Autodesk Fusion 360 part; units mm, degrees
(part 3 of 8)
  line L1878 (6.35, -70.8501) -> (9.35, -70.8501)
  line L1879 (9.35, -70.8501) -> (9.35, -67.8501)
  line L1880 (9.35, -67.8501) -> (6.35, -67.8501)
  line L1881 (6.35, -67.8501) -> (6.35, -64.8501)
  line L1882 (6.35, -64.8501) -> (9.35, -64.8501)
  line L1883 (9.35, -64.8501) -> (9.35, -61.8501)
  line L1884 (9.35, -61.8501) -> (6.35, -61.8501)
  line L1885 (6.35, -61.8501) -> (6.35, -58.85)
  line L1886 (6.35, -58.85) -> (9.35, -58.85)
  line L1887 (9.35, -58.85) -> (9.35, -55.85)
  line L1888 (9.35, -55.85) -> (6.35, -55.85)
  line L1889 (6.35, -55.85) -> (6.35, -52.85)
  line L1890 (6.35, -52.85) -> (9.35, -52.85)
  line L1891 (9.35, -52.85) -> (9.35, -49.85)
  line L1892 (9.35, -49.85) -> (6.35, -49.85)
  line L1893 (6.35, -49.85) -> (6.35, -46.85)
  line L1894 (6.35, -46.85) -> (9.35, -46.85)
  line L1895 (9.35, -46.85) -> (9.35, -43.85)
  line L1896 (9.35, -43.85) -> (6.35, -43.85)
  line L1897 (6.35, -43.85) -> (6.35, -40.85)
  line L1898 (6.35, -40.85) -> (9.35, -40.85)
  line L1899 (9.35, -40.85) -> (9.35, -37.85)
  line L1900 (9.35, -37.85) -> (6.35, -37.85)
  line L1901 (6.35, -37.85) -> (6.35, -34.85)
  line L1902 (6.35, -34.85) -> (9.35, -34.85)
  line L1903 (9.35, -34.85) -> (9.35, -31.85)
  line L1904 (9.35, -31.85) -> (6.35, -31.85)
  line L1905 (6.35, -31.85) -> (6.35, -28.1)
  line L1906 (6.35, -28.1) -> (9.35, -28.1)
  line L1907 (9.35, -28.1) -> (9.35, -27.35)
  line L1908 (325.3503, -27.35) -> (327.1003, -27.35)
  line L1909 (327.1003, -27.35) -> (327.1003, -24.35)
  line L1910 (327.1003, -24.35) -> (331.8503, -24.35)
  line L1911 (331.8503, -24.35) -> (331.8503, -27.35)
  line L1912 (331.8503, -27.35) -> (334.8503, -27.35)
  line L1913 (334.8503, -27.35) -> (334.8503, -24.35)
  line L1914 (334.8503, -24.35) -> (337.8503, -24.35)
  line L1915 (337.8503, -24.35) -> (337.8503, -27.35)
  line L1916 (337.8503, -27.35) -> (340.8503, -27.35)
  line L1917 (340.8503, -27.35) -> (340.8503, -24.35)
  line L1918 (340.8503, -24.35) -> (343.8503, -24.35)
  line L1919 (343.8503, -24.35) -> (343.8503, -27.35)
  line L1920 (343.8503, -27.35) -> (346.8503, -27.35)
  line L1921 (346.8503, -27.35) -> (346.8503, -24.35)
  line L1922 (346.8503, -24.35) -> (349.8503, -24.35)
  line L1923 (349.8503, -24.35) -> (349.8503, -27.35)
  line L1924 (349.8503, -27.35) -> (352.8503, -27.35)
  line L1925 (352.8503, -27.35) -> (352.8503, -24.35)
  line L1926 (352.8503, -24.35) -> (355.8503, -24.35)
  line L1927 (355.8503, -24.35) -> (355.8503, -27.35)
  line L1928 (355.8503, -27.35) -> (358.8503, -27.35)
  line L1929 (358.8503, -27.35) -> (358.8503, -24.35)
  line L1930 (358.8503, -24.35) -> (361.8503, -24.35)
  line L1931 (361.8503, -24.35) -> (361.8503, -27.35)
  line L1932 (361.8503, -27.35) -> (364.8503, -27.35)
  line L1933 (364.8503, -27.35) -> (364.8503, -24.35)
  line L1934 (364.8503, -24.35) -> (367.8503, -24.35)
  line L1935 (367.8503, -24.35) -> (367.8503, -27.35)
  line L1936 (367.8503, -27.35) -> (370.8503, -27.35)
  line L1937 (370.8503, -27.35) -> (370.8503, -24.35)
  line L1938 (370.8503, -24.35) -> (373.8503, -24.35)
  line L1939 (373.8503, -24.35) -> (373.8503, -27.35)
  line L1940 (373.8503, -27.35) -> (376.8503, -27.35)
  line L1941 (376.8503, -27.35) -> (376.8503, -24.35)
  line L1942 (376.8503, -24.35) -> (379.8503, -24.35)
  line L1943 (379.8503, -24.35) -> (379.8503, -27.35)
  line L1944 (379.8503, -27.35) -> (382.8503, -27.35)
  line L1945 (382.8503, -27.35) -> (382.8503, -24.35)
  line L1946 (382.8503, -24.35) -> (385.8503, -24.35)
  line L1947 (385.8503, -24.35) -> (385.8503, -27.35)
  line L1948 (385.8503, -27.35) -> (388.8503, -27.35)
  line L1949 (388.8503, -27.35) -> (388.8503, -24.35)
  line L1950 (388.8503, -24.35) -> (391.8503, -24.35)
  line L1951 (391.8503, -24.35) -> (391.8503, -27.35)
  line L1952 (391.8503, -27.35) -> (394.8503, -27.35)
  line L1953 (394.8503, -27.35) -> (394.8503, -24.35)
  line L1954 (394.8503, -24.35) -> (397.8503, -24.35)
  line L1955 (397.8503, -24.35) -> (397.8503, -27.35)
  line L1956 (397.8503, -27.35) -> (400.8503, -27.35)
  line L1957 (400.8503, -27.35) -> (400.8503, -24.35)
  line L1958 (400.8503, -24.35) -> (403.8503, -24.35)
  line L1959 (403.8503, -24.35) -> (403.8503, -27.35)
  line L1960 (403.8503, -27.35) -> (406.8503, -27.35)
  line L1961 (406.8503, -27.35) -> (406.8503, -24.35)
  line L1962 (406.8503, -24.35) -> (409.8503, -24.35)
  line L1963 (409.8503, -24.35) -> (409.8503, -27.35)
  line L1964 (409.8503, -27.35) -> (412.8503, -27.35)
  line L1965 (412.8503, -27.35) -> (412.8503, -24.35)
  line L1966 (412.8503, -24.35) -> (415.8503, -24.35)
  line L1967 (415.8503, -24.35) -> (415.8503, -27.35)
  line L1968 (415.8503, -27.35) -> (418.8503, -27.35)
  line L1969 (418.8503, -27.35) -> (418.8503, -24.35)
  line L1970 (418.8503, -24.35) -> (421.8503, -24.35)
  line L1971 (421.8503, -24.35) -> (421.8503, -27.35)
  line L1972 (421.8503, -27.35) -> (424.8503, -27.35)
  line L1973 (424.8503, -27.35) -> (424.8503, -24.35)
  line L1974 (424.8503, -24.35) -> (427.8504, -24.35)
  line L1975 (427.8504, -24.35) -> (427.8504, -27.35)
  line L1976 (427.8504, -27.35) -> (430.8504, -27.35)
  line L1977 (430.8504, -27.35) -> (430.8504, -24.35)
  line L1978 (430.8504, -24.35) -> (433.8504, -24.35)
  line L1979 (433.8504, -24.35) -> (433.8504, -27.35)
  line L1980 (433.8504, -27.35) -> (436.8504, -27.35)
  line L1981 (436.8504, -27.35) -> (436.8504, -24.35)
  line L1982 (436.8504, -24.35) -> (439.8504, -24.35)
  line L1983 (439.8504, -24.35) -> (439.8504, -27.35)
  line L1984 (439.8504, -27.35) -> (442.8504, -27.35)
  line L1985 (442.8504, -27.35) -> (442.8504, -24.35)
  line L1986 (442.8504, -24.35) -> (445.8504, -24.35)
  line L1987 (445.8504, -24.35) -> (445.8504, -27.35)
  line L1988 (445.8504, -27.35) -> (448.8504, -27.35)
  line L1989 (448.8504, -27.35) -> (448.8504, -24.35)
  line L1990 (448.8504, -24.35) -> (451.8504, -24.35)
  line L1991 (451.8504, -24.35) -> (451.8504, -27.35)
  line L1992 (451.8504, -27.35) -> (454.8504, -27.35)
  line L1993 (454.8504, -27.35) -> (454.8504, -24.35)
  line L1994 (454.8504, -24.35) -> (457.8504, -24.35)
  line L1995 (457.8504, -24.35) -> (457.8504, -27.35)
  line L1996 (457.8504, -27.35) -> (460.8504, -27.35)
  line L1997 (460.8504, -27.35) -> (460.8504, -24.35)
  line L1998 (460.8504, -24.35) -> (463.8504, -24.35)
  line L1999 (463.8504, -24.35) -> (463.8504, -27.35)
  line L2000 (463.8504, -27.35) -> (466.8504, -27.35)
  line L2001 (466.8504, -27.35) -> (466.8504, -24.35)
  line L2002 (466.8504, -24.35) -> (469.8504, -24.35)
  line L2003 (469.8504, -24.35) -> (469.8504, -27.35)
  line L2004 (469.8504, -27.35) -> (472.8504, -27.35)
  line L2005 (472.8504, -27.35) -> (472.8504, -24.35)
  line L2006 (472.8504, -24.35) -> (475.8504, -24.35)
  line L2007 (475.8504, -24.35) -> (475.8504, -27.35)
  line L2008 (475.8504, -27.35) -> (478.8504, -27.35)
  line L2009 (478.8504, -27.35) -> (478.8504, -24.35)
  line L2010 (478.8504, -24.35) -> (481.8504, -24.35)
  line L2011 (481.8504, -24.35) -> (481.8504, -27.35)
  line L2012 (481.8504, -27.35) -> (484.8504, -27.35)
  line L2013 (484.8504, -27.35) -> (484.8504, -24.35)
  line L2014 (484.8504, -24.35) -> (487.8504, -24.35)
  line L2015 (487.8504, -24.35) -> (487.8504, -27.35)
  line L2016 (487.8504, -27.35) -> (490.8504, -27.35)
  line L2017 (490.8504, -27.35) -> (490.8504, -24.35)
  line L2018 (490.8504, -24.35) -> (493.8504, -24.35)
  line L2019 (493.8504, -24.35) -> (493.8504, -27.35)
  line L2020 (493.8504, -27.35) -> (496.8504, -27.35)
  line L2021 (496.8504, -27.35) -> (496.8504, -24.35)
  line L2022 (496.8504, -24.35) -> (499.8504, -24.35)
  line L2023 (499.8504, -24.35) -> (499.8504, -27.35)
  line L2024 (499.8504, -27.35) -> (502.8504, -27.35)
  line L2025 (502.8504, -27.35) -> (502.8504, -24.35)
  line L2026 (502.8504, -24.35) -> (505.8504, -24.35)
  line L2027 (505.8504, -24.35) -> (505.8504, -27.35)
  line L2028 (505.8504, -27.35) -> (508.8504, -27.35)
  line L2029 (508.8504, -27.35) -> (508.8504, -24.35)
  line L2030 (508.8504, -24.35) -> (511.8504, -24.35)
  line L2031 (511.8504, -24.35) -> (511.8504, -27.35)
  line L2032 (511.8504, -27.35) -> (514.8504, -27.35)
  line L2033 (514.8504, -27.35) -> (514.8504, -24.35)
  line L2034 (514.8504, -24.35) -> (517.8504, -24.35)
  line L2035 (517.8504, -24.35) -> (517.8504, -27.35)
  line L2036 (517.8504, -27.35) -> (520.8504, -27.35)
  line L2037 (520.8504, -27.35) -> (520.8504, -24.35)
  line L2038 (520.8504, -24.35) -> (523.8504, -24.35)
  line L2039 (523.8504, -24.35) -> (523.8504, -27.35)
  line L2040 (523.8504, -27.35) -> (526.8504, -27.35)
  line L2041 (526.8504, -27.35) -> (526.8504, -24.35)
  line L2042 (526.8504, -24.35) -> (529.8504, -24.35)
  line L2043 (529.8504, -24.35) -> (529.8504, -27.35)
  line L2044 (529.8504, -27.35) -> (532.8504, -27.35)
  line L2045 (532.8504, -27.35) -> (532.8504, -24.35)
  line L2046 (532.8504, -24.35) -> (535.8504, -24.35)
  line L2047 (535.8504, -24.35) -> (535.8504, -27.35)
  line L2048 (535.8504, -27.35) -> (538.8504, -27.35)
  line L2049 (538.8504, -27.35) -> (538.8504, -24.35)
  line L2050 (538.8504, -24.35) -> (541.8504, -24.35)
  line L2051 (541.8504, -24.35) -> (541.8504, -27.35)
  line L2052 (541.8504, -27.35) -> (544.8504, -27.35)
  line L2053 (544.8504, -27.35) -> (544.8504, -24.35)
  line L2054 (544.8504, -24.35) -> (547.8505, -24.35)
  line L2055 (547.8505, -24.35) -> (547.8505, -27.35)
  line L2056 (547.8505, -27.35) -> (550.8505, -27.35)
  line L2057 (550.8505, -27.35) -> (550.8505, -24.35)
  line L2058 (550.8505, -24.35) -> (553.8505, -24.35)
  line L2059 (553.8505, -24.35) -> (553.8505, -27.35)
  line L2060 (553.8505, -27.35) -> (556.8505, -27.35)
  line L2061 (556.8505, -27.35) -> (556.8505, -24.35)
  line L2062 (556.8505, -24.35) -> (559.8505, -24.35)
  line L2063 (559.8505, -24.35) -> (559.8505, -27.35)
  line L2064 (559.8505, -27.35) -> (562.8505, -27.35)
  line L2065 (562.8505, -27.35) -> (562.8505, -24.35)
  line L2066 (562.8505, -24.35) -> (565.8505, -24.35)
  line L2067 (565.8505, -24.35) -> (565.8505, -27.35)
  line L2068 (565.8505, -27.35) -> (568.8505, -27.35)
  line L2069 (568.8505, -27.35) -> (568.8505, -24.35)
  line L2070 (568.8505, -24.35) -> (571.8505, -24.35)
  line L2071 (571.8505, -24.35) -> (571.8505, -27.35)
  line L2072 (571.8505, -27.35) -> (574.8505, -27.35)
  line L2073 (574.8505, -27.35) -> (574.8505, -24.35)
  line L2074 (574.8505, -24.35) -> (577.8505, -24.35)
  line L2075 (577.8505, -24.35) -> (577.8505, -27.35)
  line L2076 (577.8505, -27.35) -> (580.8505, -27.35)
  line L2077 (580.8505, -27.35) -> (580.8505, -24.35)
  line L2078 (580.8505, -24.35) -> (583.8505, -24.35)
  line L2079 (583.8505, -24.35) -> (583.8505, -27.35)
  line L2080 (583.8505, -27.35) -> (586.8505, -27.35)
  line L2081 (586.8505, -27.35) -> (586.8505, -24.35)
  line L2082 (586.8505, -24.35) -> (589.8505, -24.35)
  line L2083 (589.8505, -24.35) -> (589.8505, -27.35)
  line L2084 (589.8505, -27.35) -> (592.8505, -27.35)
  line L2085 (592.8505, -27.35) -> (592.8505, -24.35)
  line L2086 (592.8505, -24.35) -> (595.8505, -24.35)
  line L2087 (595.8505, -24.35) -> (595.8505, -27.35)
  line L2088 (595.8505, -27.35) -> (598.8505, -27.35)
  line L2089 (598.8505, -27.35) -> (598.8505, -24.35)
  line L2090 (598.8505, -24.35) -> (601.8505, -24.35)
  line L2091 (601.8505, -24.35) -> (601.8505, -27.35)
  line L2092 (601.8505, -27.35) -> (604.8505, -27.35)
  line L2093 (604.8505, -27.35) -> (604.8505, -24.35)
  line L2094 (604.8505, -24.35) -> (607.8505, -24.35)
  line L2095 (607.8505, -24.35) -> (607.8505, -27.35)
  line L2096 (607.8505, -27.35) -> (610.8505, -27.35)
  line L2097 (610.8505, -27.35) -> (610.8505, -24.35)
  line L2098 (610.8505, -24.35) -> (613.8505, -24.35)
  line L2099 (613.8505, -24.35) -> (613.8505, -27.35)
  line L2100 (613.8505, -27.35) -> (616.8505, -27.35)
  line L2101 (616.8505, -27.35) -> (616.8505, -24.35)
  line L2102 (616.8505, -24.35) -> (619.8505, -24.35)
  line L2103 (619.8505, -24.35) -> (619.8505, -27.35)
  line L2104 (619.8505, -27.35) -> (622.8505, -27.35)
  line L2105 (622.8505, -27.35) -> (622.8505, -24.35)
  line L2106 (622.8505, -24.35) -> (625.8505, -24.35)
  line L2107 (625.8505, -24.35) -> (625.8505, -27.35)
  line L2108 (625.8505, -27.35) -> (628.8505, -27.35)
  line L2109 (628.8505, -27.35) -> (628.8505, -24.35)
  line L2110 (628.8505, -24.35) -> (633.6005, -24.35)
  line L2111 (633.6005, -24.35) -> (633.6005, -27.35)
  line L2112 (633.6005, -27.35) -> (635.3505, -27.35)
  line L2113 (635.3505, -27.35) -> (635.3505, -28.1)
  line L2114 (635.3505, -28.1) -> (638.3505, -28.1)
  line L2115 (638.3505, -28.1) -> (638.3505, -31.85)
  line L2116 (638.3505, -31.85) -> (635.3505, -31.85)
  line L2117 (635.3505, -31.85) -> (635.3505, -34.85)
  line L2118 (635.3505, -34.85) -> (638.3505, -34.85)
  line L2119 (638.3505, -34.85) -> (638.3505, -37.85)
  line L2120 (638.3505, -37.85) -> (635.3505, -37.85)
  line L2121 (635.3505, -37.85) -> (635.3505, -40.85)
  line L2122 (635.3505, -40.85) -> (638.3505, -40.85)
  line L2123 (638.3505, -40.85) -> (638.3505, -43.85)
  line L2124 (638.3505, -43.85) -> (635.3505, -43.85)
  line L2125 (635.3505, -43.85) -> (635.3505, -46.85)
  line L2126 (635.3505, -46.85) -> (638.3505, -46.85)
  line L2127 (638.3505, -46.85) -> (638.3505, -49.85)
  line L2128 (638.3505, -49.85) -> (635.3505, -49.85)
  line L2129 (635.3505, -49.85) -> (635.3505, -52.85)
  line L2130 (635.3505, -52.85) -> (638.3505, -52.85)
  line L2131 (638.3505, -52.85) -> (638.3505, -55.85)
  line L2132 (638.3505, -55.85) -> (635.3505, -55.85)
  line L2133 (635.3505, -55.85) -> (635.3505, -58.85)
  line L2134 (635.3505, -58.85) -> (638.3505, -58.85)
  line L2135 (638.3505, -58.85) -> (638.3505, -61.8501)
  line L2136 (638.3505, -61.8501) -> (635.3505, -61.8501)
  line L2137 (635.3505, -61.8501) -> (635.3505, -64.8501)
  line L2138 (635.3505, -64.8501) -> (638.3505, -64.8501)
  line L2139 (638.3505, -64.8501) -> (638.3505, -67.8501)
  line L2140 (638.3505, -67.8501) -> (635.3505, -67.8501)
  line L2141 (635.3505, -67.8501) -> (635.3505, -70.8501)
  line L2142 (635.3505, -70.8501) -> (638.3505, -70.8501)
  line L2143 (638.3505, -70.8501) -> (638.3505, -73.8501)
  line L2144 (638.3505, -73.8501) -> (635.3505, -73.8501)
  line L2145 (635.3505, -73.8501) -> (635.3505, -76.8501)
  line L2146 (635.3505, -76.8501) -> (638.3505, -76.8501)
  line L2147 (638.3505, -76.8501) -> (638.3505, -79.8501)
  line L2148 (638.3505, -79.8501) -> (635.3505, -79.8501)
  line L2149 (635.3505, -79.8501) -> (635.3505, -82.8501)
  line L2150 (635.3505, -82.8501) -> (638.3505, -82.8501)
  line L2151 (638.3505, -82.8501) -> (638.3505, -85.8501)
  line L2152 (638.3505, -85.8501) -> (635.3505, -85.8501)
  line L2153 (635.3505, -85.8501) -> (635.3505, -88.8501)
  line L2154 (635.3505, -88.8501) -> (638.3505, -88.8501)
  line L2155 (638.3505, -88.8501) -> (638.3505, -91.8501)
  line L2156 (638.3505, -91.8501) -> (635.3505, -91.8501)
  line L2157 (635.3505, -91.8501) -> (635.3505, -94.8501)
  line L2158 (635.3505, -94.8501) -> (638.3505, -94.8501)
  line L2159 (638.3505, -94.8501) -> (638.3505, -97.8501)
  line L2160 (638.3505, -97.8501) -> (635.3505, -97.8501)
  line L2161 (635.3505, -97.8501) -> (635.3505, -100.8501)
  line L2162 (635.3505, -100.8501) -> (638.3505, -100.8501)
  line L2163 (638.3505, -100.8501) -> (638.3505, -103.8501)
  line L2164 (638.3505, -103.8501) -> (635.3505, -103.8501)
  line L2165 (635.3505, -103.8501) -> (635.3505, -106.8501)
  line L2166 (635.3505, -106.8501) -> (638.3505, -106.8501)
  line L2167 (638.3505, -106.8501) -> (638.3505, -109.8501)
  line L2168 (638.3505, -109.8501) -> (635.3505, -109.8501)
  line L2169 (635.3505, -109.8501) -> (635.3505, -112.8501)
  line L2170 (635.3505, -112.8501) -> (638.3505, -112.8501)
  line L2171 (638.3505, -112.8501) -> (638.3505, -115.8501)
  line L2172 (638.3505, -115.8501) -> (635.3505, -115.8501)
  line L2173 (635.3505, -115.8501) -> (635.3505, -118.8501)
  line L2174 (635.3505, -118.8501) -> (638.3505, -118.8501)
  line L2175 (638.3505, -118.8501) -> (638.3505, -121.8501)
  line L2176 (638.3505, -121.8501) -> (635.3505, -121.8501)
  line L2177 (635.3505, -121.8501) -> (635.3505, -124.8501)
  line L2178 (635.3505, -124.8501) -> (638.3505, -124.8501)
  line L2179 (638.3505, -124.8501) -> (638.3505, -127.8501)
  line L2180 (638.3505, -127.8501) -> (635.3505, -127.8501)
  line L2181 (635.3505, -127.8501) -> (635.3505, -130.8501)
  line L2182 (635.3505, -130.8501) -> (638.3505, -130.8501)
  line L2183 (638.3505, -130.8501) -> (638.3505, -133.8501)
  line L2184 (638.3505, -133.8501) -> (635.3505, -133.8501)
  line L2185 (635.3505, -133.8501) -> (635.3505, -136.8501)
  line L2186 (635.3505, -136.8501) -> (638.3505, -136.8501)
  line L2187 (638.3505, -136.8501) -> (638.3505, -139.8501)
  line L2188 (638.3505, -139.8501) -> (635.3505, -139.8501)
  line L2189 (635.3505, -139.8501) -> (635.3505, -142.8501)
  line L2190 (635.3505, -142.8501) -> (638.3505, -142.8501)
  line L2191 (638.3505, -142.8501) -> (638.3505, -145.8501)
  line L2192 (638.3505, -145.8501) -> (635.3505, -145.8501)
  line L2193 (635.3505, -145.8501) -> (635.3505, -148.8501)
  line L2194 (635.3505, -148.8501) -> (638.3505, -148.8501)
  line L2195 (638.3505, -148.8501) -> (638.3505, -151.8501)
  line L2196 (638.3505, -151.8501) -> (635.3505, -151.8501)
  line L2197 (635.3505, -151.8501) -> (635.3505, -154.8501)
  line L2198 (635.3505, -154.8501) -> (638.3505, -154.8501)
  line L2199 (638.3505, -154.8501) -> (638.3505, -157.8501)
  line L2200 (638.3505, -157.8501) -> (635.3505, -157.8501)
  line L2201 (635.3505, -157.8501) -> (635.3505, -160.8501)
  line L2202 (635.3505, -160.8501) -> (638.3505, -160.8501)
  line L2203 (638.3505, -160.8501) -> (638.3505, -163.8501)
  line L2204 (638.3505, -163.8501) -> (635.3505, -163.8501)
  line L2205 (635.3505, -163.8501) -> (635.3505, -166.8501)
  line L2206 (635.3505, -166.8501) -> (638.3505, -166.8501)
  line L2207 (638.3505, -166.8501) -> (638.3505, -169.8501)
  line L2208 (638.3505, -169.8501) -> (635.3505, -169.8501)
  line L2209 (635.3505, -169.8501) -> (635.3505, -172.8501)
  line L2210 (635.3505, -172.8501) -> (638.3505, -172.8501)
  line L2211 (638.3505, -172.8501) -> (638.3505, -176.6001)
  line L2212 (638.3505, -176.6001) -> (635.3505, -176.6001)
  line L2213 (635.3505, -176.6001) -> (635.3505, -177.3501)
  line L2214 (635.3505, -177.3501) -> (633.6005, -177.3501)
  line L2215 (633.6005, -177.3501) -> (633.6005, -180.3501)
  line L2216 (633.6005, -180.3501) -> (628.8505, -180.3501)
  line L2217 (628.8505, -180.3501) -> (628.8505, -177.3501)
  line L2218 (628.8505, -177.3501) -> (625.8505, -177.3501)
  line L2219 (625.8505, -177.3501) -> (625.8505, -180.3501)
  line L2220 (625.8505, -180.3501) -> (622.8505, -180.3501)
  line L2221 (622.8505, -180.3501) -> (622.8505, -177.3501)
  line L2222 (622.8505, -177.3501) -> (619.8505, -177.3501)
  line L2223 (619.8505, -177.3501) -> (619.8505, -180.3501)
  line L2224 (619.8505, -180.3501) -> (616.8505, -180.3501)
  line L2225 (616.8505, -180.3501) -> (616.8505, -177.3501)
  line L2226 (616.8505, -177.3501) -> (613.8505, -177.3501)
  line L2227 (613.8505, -177.3501) -> (613.8505, -180.3501)
  line L2228 (613.8505, -180.3501) -> (610.8505, -180.3501)
  line L2229 (610.8505, -180.3501) -> (610.8505, -177.3501)
  line L2230 (610.8505, -177.3501) -> (607.8505, -177.3501)
  line L2231 (607.8505, -177.3501) -> (607.8505, -180.3501)
  line L2232 (607.8505, -180.3501) -> (604.8505, -180.3501)
  line L2233 (604.8505, -180.3501) -> (604.8505, -177.3501)
  line L2234 (604.8505, -177.3501) -> (601.8505, -177.3501)
  line L2235 (601.8505, -177.3501) -> (601.8505, -180.3501)
  line L2236 (601.8505, -180.3501) -> (598.8505, -180.3501)
  line L2237 (598.8505, -180.3501) -> (598.8505, -177.3501)
  line L2238 (598.8505, -177.3501) -> (595.8505, -177.3501)
  line L2239 (595.8505, -177.3501) -> (595.8505, -180.3501)
  line L2240 (595.8505, -180.3501) -> (592.8505, -180.3501)
  line L2241 (592.8505, -180.3501) -> (592.8505, -177.3501)
  line L2242 (592.8505, -177.3501) -> (589.8505, -177.3501)
  line L2243 (589.8505, -177.3501) -> (589.8505, -180.3501)
  line L2244 (589.8505, -180.3501) -> (586.8505, -180.3501)
  line L2245 (586.8505, -180.3501) -> (586.8505, -177.3501)
  line L2246 (586.8505, -177.3501) -> (583.8505, -177.3501)
  line L2247 (583.8505, -177.3501) -> (583.8505, -180.3501)
  line L2248 (583.8505, -180.3501) -> (580.8505, -180.3501)
  line L2249 (580.8505, -180.3501) -> (580.8505, -177.3501)
  line L2250 (580.8505, -177.3501) -> (577.8505, -177.3501)
  line L2251 (577.8505, -177.3501) -> (577.8505, -180.3501)
  line L2252 (577.8505, -180.3501) -> (574.8505, -180.3501)
  line L2253 (574.8505, -180.3501) -> (574.8505, -177.3501)
  line L2254 (574.8505, -177.3501) -> (571.8505, -177.3501)
  line L2255 (571.8505, -177.3501) -> (571.8505, -180.3501)
  line L2256 (571.8505, -180.3501) -> (568.8505, -180.3501)
  line L2257 (568.8505, -180.3501) -> (568.8505, -177.3501)
  line L2258 (568.8505, -177.3501) -> (565.8505, -177.3501)
  line L2259 (565.8505, -177.3501) -> (565.8505, -180.3501)
  line L2260 (565.8505, -180.3501) -> (562.8505, -180.3501)
  line L2261 (562.8505, -180.3501) -> (562.8505, -177.3501)
  line L2262 (562.8505, -177.3501) -> (559.8505, -177.3501)
  line L2263 (559.8505, -177.3501) -> (559.8505, -180.3501)
  line L2264 (559.8505, -180.3501) -> (556.8505, -180.3501)
  line L2265 (556.8505, -180.3501) -> (556.8505, -177.3501)
  line L2266 (556.8505, -177.3501) -> (553.8505, -177.3501)
  line L2267 (553.8505, -177.3501) -> (553.8505, -180.3501)
  line L2268 (553.8505, -180.3501) -> (550.8505, -180.3501)
  line L2269 (550.8505, -180.3501) -> (550.8505, -177.3501)
  line L2270 (550.8505, -177.3501) -> (547.8505, -177.3501)
  line L2271 (547.8505, -177.3501) -> (547.8505, -180.3501)
  line L2272 (547.8505, -180.3501) -> (544.8504, -180.3501)
  line L2273 (544.8504, -180.3501) -> (544.8504, -177.3501)
  line L2274 (544.8504, -177.3501) -> (541.8504, -177.3501)
  line L2275 (541.8504, -177.3501) -> (541.8504, -180.3501)
  line L2276 (541.8504, -180.3501) -> (538.8504, -180.3501)
  line L2277 (538.8504, -180.3501) -> (538.8504, -177.3501)
  line L2278 (538.8504, -177.3501) -> (535.8504, -177.3501)
  line L2279 (535.8504, -177.3501) -> (535.8504, -180.3501)
  line L2280 (535.8504, -180.3501) -> (532.8504, -180.3501)
  line L2281 (532.8504, -180.3501) -> (532.8504, -177.3501)
  line L2282 (532.8504, -177.3501) -> (529.8504, -177.3501)
  line L2283 (529.8504, -177.3501) -> (529.8504, -180.3501)
  line L2284 (529.8504, -180.3501) -> (526.8504, -180.3501)
  line L2285 (526.8504, -180.3501) -> (526.8504, -177.3501)
  line L2286 (526.8504, -177.3501) -> (523.8504, -177.3501)
  line L2287 (523.8504, -177.3501) -> (523.8504, -180.3501)
  line L2288 (523.8504, -180.3501) -> (520.8504, -180.3501)
  line L2289 (520.8504, -180.3501) -> (520.8504, -177.3501)
  line L2290 (520.8504, -177.3501) -> (517.8504, -177.3501)
  line L2291 (517.8504, -177.3501) -> (517.8504, -180.3501)
  line L2292 (517.8504, -180.3501) -> (514.8504, -180.3501)
  line L2293 (514.8504, -180.3501) -> (514.8504, -177.3501)
  line L2294 (514.8504, -177.3501) -> (511.8504, -177.3501)
  line L2295 (511.8504, -177.3501) -> (511.8504, -180.3501)
  line L2296 (511.8504, -180.3501) -> (508.8504, -180.3501)
  line L2297 (508.8504, -180.3501) -> (508.8504, -177.3501)
  line L2298 (508.8504, -177.3501) -> (505.8504, -177.3501)
  line L2299 (505.8504, -177.3501) -> (505.8504, -180.3501)
  line L2300 (505.8504, -180.3501) -> (502.8504, -180.3501)
  line L2301 (502.8504, -180.3501) -> (502.8504, -177.3501)
  line L2302 (502.8504, -177.3501) -> (499.8504, -177.3501)
  line L2303 (499.8504, -177.3501) -> (499.8504, -180.3501)
  line L2304 (499.8504, -180.3501) -> (496.8504, -180.3501)
  line L2305 (496.8504, -180.3501) -> (496.8504, -177.3501)
  line L2306 (496.8504, -177.3501) -> (493.8504, -177.3501)
  line L2307 (493.8504, -177.3501) -> (493.8504, -180.3501)
  line L2308 (493.8504, -180.3501) -> (490.8504, -180.3501)
  line L2309 (490.8504, -180.3501) -> (490.8504, -177.3501)
  line L2310 (490.8504, -177.3501) -> (487.8504, -177.3501)
  line L2311 (487.8504, -177.3501) -> (487.8504, -180.3501)
  line L2312 (487.8504, -180.3501) -> (484.8504, -180.3501)
  line L2313 (484.8504, -180.3501) -> (484.8504, -177.3501)
  line L2314 (484.8504, -177.3501) -> (481.8504, -177.3501)
  line L2315 (481.8504, -177.3501) -> (481.8504, -180.3501)
  line L2316 (481.8504, -180.3501) -> (478.8504, -180.3501)
  line L2317 (478.8504, -180.3501) -> (478.8504, -177.3501)
  line L2318 (478.8504, -177.3501) -> (475.8504, -177.3501)
  line L2319 (475.8504, -177.3501) -> (475.8504, -180.3501)
  line L2320 (475.8504, -180.3501) -> (472.8504, -180.3501)
  line L2321 (472.8504, -180.3501) -> (472.8504, -177.3501)
  line L2322 (472.8504, -177.3501) -> (469.8504, -177.3501)
  line L2323 (469.8504, -177.3501) -> (469.8504, -180.3501)
  line L2324 (469.8504, -180.3501) -> (466.8504, -180.3501)
  line L2325 (466.8504, -180.3501) -> (466.8504, -177.3501)
  line L2326 (466.8504, -177.3501) -> (463.8504, -177.3501)
  line L2327 (463.8504, -177.3501) -> (463.8504, -180.3501)
  line L2328 (463.8504, -180.3501) -> (460.8504, -180.3501)
  line L2329 (460.8504, -180.3501) -> (460.8504, -177.3501)
  line L2330 (460.8504, -177.3501) -> (457.8504, -177.3501)
  line L2331 (457.8504, -177.3501) -> (457.8504, -180.3501)
  line L2332 (457.8504, -180.3501) -> (454.8504, -180.3501)
  line L2333 (454.8504, -180.3501) -> (454.8504, -177.3501)
  line L2334 (454.8504, -177.3501) -> (451.8504, -177.3501)
  line L2335 (451.8504, -177.3501) -> (451.8504, -180.3501)
  line L2336 (451.8504, -180.3501) -> (448.8504, -180.3501)
  line L2337 (448.8504, -180.3501) -> (448.8504, -177.3501)
  line L2338 (448.8504, -177.3501) -> (445.8504, -177.3501)
  line L2339 (445.8504, -177.3501) -> (445.8504, -180.3501)
  line L2340 (445.8504, -180.3501) -> (442.8504, -180.3501)
  line L2341 (442.8504, -180.3501) -> (442.8504, -177.3501)
  line L2342 (442.8504, -177.3501) -> (439.8504, -177.3501)
  line L2343 (439.8504, -177.3501) -> (439.8504, -180.3501)
  line L2344 (439.8504, -180.3501) -> (436.8504, -180.3501)
  line L2345 (436.8504, -180.3501) -> (436.8504, -177.3501)
  line L2346 (436.8504, -177.3501) -> (433.8504, -177.3501)
  line L2347 (433.8504, -177.3501) -> (433.8504, -180.3501)
  line L2348 (433.8504, -180.3501) -> (430.8504, -180.3501)
  line L2349 (430.8504, -180.3501) -> (430.8504, -177.3501)
  line L2350 (430.8504, -177.3501) -> (427.8504, -177.3501)
  line L2351 (427.8504, -177.3501) -> (427.8504, -180.3501)
  line L2352 (427.8504, -180.3501) -> (424.8503, -180.3501)
  line L2353 (424.8503, -180.3501) -> (424.8503, -177.3501)
  line L2354 (424.8503, -177.3501) -> (421.8503, -177.3501)
  line L2355 (421.8503, -177.3501) -> (421.8503, -180.3501)
  line L2356 (421.8503, -180.3501) -> (418.8503, -180.3501)
  line L2357 (418.8503, -180.3501) -> (418.8503, -177.3501)
  line L2358 (418.8503, -177.3501) -> (415.8503, -177.3501)
  line L2359 (415.8503, -177.3501) -> (415.8503, -180.3501)
  line L2360 (415.8503, -180.3501) -> (412.8503, -180.3501)
  line L2361 (412.8503, -180.3501) -> (412.8503, -177.3501)
  line L2362 (412.8503, -177.3501) -> (409.8503, -177.3501)
  line L2363 (409.8503, -177.3501) -> (409.8503, -180.3501)
  line L2364 (409.8503, -180.3501) -> (406.8503, -180.3501)
  line L2365 (406.8503, -180.3501) -> (406.8503, -177.3501)
  line L2366 (406.8503, -177.3501) -> (403.8503, -177.3501)
  line L2367 (403.8503, -177.3501) -> (403.8503, -180.3501)
  line L2368 (403.8503, -180.3501) -> (400.8503, -180.3501)
  line L2369 (400.8503, -180.3501) -> (400.8503, -177.3501)
  line L2370 (400.8503, -177.3501) -> (397.8503, -177.3501)
  line L2371 (397.8503, -177.3501) -> (397.8503, -180.3501)
  line L2372 (397.8503, -180.3501) -> (394.8503, -180.3501)
  line L2373 (394.8503, -180.3501) -> (394.8503, -177.3501)
  line L2374 (394.8503, -177.3501) -> (391.8503, -177.3501)
  line L2375 (391.8503, -177.3501) -> (391.8503, -180.3501)
  line L2376 (391.8503, -180.3501) -> (388.8503, -180.3501)
  line L2377 (388.8503, -180.3501) -> (388.8503, -177.3501)
  line L2378 (388.8503, -177.3501) -> (385.8503, -177.3501)
  line L2379 (385.8503, -177.3501) -> (385.8503, -180.3501)
  line L2380 (385.8503, -180.3501) -> (382.8503, -180.3501)
  line L2381 (382.8503, -180.3501) -> (382.8503, -177.3501)
  line L2382 (382.8503, -177.3501) -> (379.8503, -177.3501)
  line L2383 (379.8503, -177.3501) -> (379.8503, -180.3501)
  line L2384 (379.8503, -180.3501) -> (376.8503, -180.3501)
  line L2385 (376.8503, -180.3501) -> (376.8503, -177.3501)
  line L2386 (376.8503, -177.3501) -> (373.8503, -177.3501)
  line L2387 (373.8503, -177.3501) -> (373.8503, -180.3501)
  line L2388 (373.8503, -180.3501) -> (370.8503, -180.3501)
  line L2389 (370.8503, -180.3501) -> (370.8503, -177.3501)
  line L2390 (370.8503, -177.3501) -> (367.8503, -177.3501)
  line L2391 (367.8503, -177.3501) -> (367.8503, -180.3501)
  line L2392 (367.8503, -180.3501) -> (364.8503, -180.3501)
  line L2393 (364.8503, -180.3501) -> (364.8503, -177.3501)
  line L2394 (364.8503, -177.3501) -> (361.8503, -177.3501)
  line L2395 (361.8503, -177.3501) -> (361.8503, -180.3501)
  line L2396 (361.8503, -180.3501) -> (358.8503, -180.3501)
  line L2397 (358.8503, -180.3501) -> (358.8503, -177.3501)
  line L2398 (358.8503, -177.3501) -> (355.8503, -177.3501)
  line L2399 (355.8503, -177.3501) -> (355.8503, -180.3501)
  line L2400 (355.8503, -180.3501) -> (352.8503, -180.3501)
  line L2401 (352.8503, -180.3501) -> (352.8503, -177.3501)
  line L2402 (352.8503, -177.3501) -> (349.8503, -177.3501)
  line L2403 (349.8503, -177.3501) -> (349.8503, -180.3501)
  line L2404 (349.8503, -180.3501) -> (346.8503, -180.3501)
  line L2405 (346.8503, -180.3501) -> (346.8503, -177.3501)
  line L2406 (346.8503, -177.3501) -> (343.8503, -177.3501)
  line L2407 (343.8503, -177.3501) -> (343.8503, -180.3501)
  line L2408 (343.8503, -180.3501) -> (340.8503, -180.3501)
  line L2409 (340.8503, -180.3501) -> (340.8503, -177.3501)
  line L2410 (340.8503, -177.3501) -> (337.8503, -177.3501)
  line L2411 (337.8503, -177.3501) -> (337.8503, -180.3501)
  line L2412 (337.8503, -180.3501) -> (334.8503, -180.3501)
  line L2413 (334.8503, -180.3501) -> (334.8503, -177.3501)
  line L2414 (334.8503, -177.3501) -> (331.8503, -177.3501)
  line L2415 (331.8503, -177.3501) -> (331.8503, -180.3501)
  line L2416 (331.8503, -180.3501) -> (327.1003, -180.3501)
  line L2417 (327.1003, -180.3501) -> (327.1003, -177.3501)
  line L2418 (327.1003, -177.3501) -> (325.3503, -177.3501)
  line L2419 (325.3503, -177.3501) -> (325.3503, -176.6001)
  line L2420 (325.3503, -176.6001) -> (322.3503, -176.6001)
  line L2421 (322.3503, -176.6001) -> (322.3503, -172.8501)
  line L2422 (322.3503, -172.8501) -> (325.3503, -172.8501)
  line L2423 (325.3503, -172.8501) -> (325.3503, -169.8501)
  line L2424 (325.3503, -169.8501) -> (322.3503, -169.8501)
  line L2425 (322.3503, -169.8501) -> (322.3503, -166.8501)
  line L2426 (322.3503, -166.8501) -> (325.3503, -166.8501)
  line L2427 (325.3503, -166.8501) -> (325.3503, -163.8501)
  line L2428 (325.3503, -163.8501) -> (322.3503, -163.8501)
  line L2429 (322.3503, -163.8501) -> (322.3503, -160.8501)
  line L2430 (322.3503, -160.8501) -> (325.3503, -160.8501)
  line L2431 (325.3503, -160.8501) -> (325.3503, -157.8501)
  line L2432 (325.3503, -157.8501) -> (322.3503, -157.8501)
  line L2433 (322.3503, -157.8501) -> (322.3503, -154.8501)
  line L2434 (322.3503, -154.8501) -> (325.3503, -154.8501)
  line L2435 (325.3503, -154.8501) -> (325.3503, -151.8501)
  line L2436 (325.3503, -151.8501) -> (322.3503, -151.8501)
  line L2437 (322.3503, -151.8501) -> (322.3503, -148.8501)
  line L2438 (322.3503, -148.8501) -> (325.3503, -148.8501)
  line L2439 (325.3503, -148.8501) -> (325.3503, -145.8501)
  line L2440 (325.3503, -145.8501) -> (322.3503, -145.8501)
  line L2441 (322.3503, -145.8501) -> (322.3503, -142.8501)
  line L2442 (322.3503, -142.8501) -> (325.3503, -142.8501)
  line L2443 (325.3503, -142.8501) -> (325.3503, -139.8501)
  line L2444 (325.3503, -139.8501) -> (322.3503, -139.8501)
  line L2445 (322.3503, -139.8501) -> (322.3503, -136.8501)
  line L2446 (322.3503, -136.8501) -> (325.3503, -136.8501)
  line L2447 (325.3503, -136.8501) -> (325.3503, -133.8501)
  line L2448 (325.3503, -133.8501) -> (322.3503, -133.8501)
  line L2449 (322.3503, -133.8501) -> (322.3503, -130.8501)
  line L2450 (322.3503, -130.8501) -> (325.3503, -130.8501)
  line L2451 (325.3503, -130.8501) -> (325.3503, -127.8501)
  line L2452 (325.3503, -127.8501) -> (322.3503, -127.8501)
  line L2453 (322.3503, -127.8501) -> (322.3503, -124.8501)
  line L2454 (322.3503, -124.8501) -> (325.3503, -124.8501)
  line L2455 (325.3503, -124.8501) -> (325.3503, -121.8501)
  line L2456 (325.3503, -121.8501) -> (322.3503, -121.8501)
  line L2457 (322.3503, -121.8501) -> (322.3503, -118.8501)
  line L2458 (322.3503, -118.8501) -> (325.3503, -118.8501)
  line L2459 (325.3503, -118.8501) -> (325.3503, -115.8501)
  line L2460 (325.3503, -115.8501) -> (322.3503, -115.8501)
  line L2461 (322.3503, -115.8501) -> (322.3503, -112.8501)
  line L2462 (322.3503, -112.8501) -> (325.3503, -112.8501)
  line L2463 (325.3503, -112.8501) -> (325.3503, -109.8501)
  line L2464 (325.3503, -109.8501) -> (322.3503, -109.8501)
  line L2465 (322.3503, -109.8501) -> (322.3503, -106.8501)
  line L2466 (322.3503, -106.8501) -> (325.3503, -106.8501)
  line L2467 (325.3503, -106.8501) -> (325.3503, -103.8501)
  line L2468 (325.3503, -103.8501) -> (322.3503, -103.8501)
  line L2469 (322.3503, -103.8501) -> (322.3503, -100.8501)
  line L2470 (322.3503, -100.8501) -> (325.3503, -100.8501)
  line L2471 (325.3503, -100.8501) -> (325.3503, -97.8501)
  line L2472 (325.3503, -97.8501) -> (322.3503, -97.8501)
  line L2473 (322.3503, -97.8501) -> (322.3503, -94.8501)
  line L2474 (322.3503, -94.8501) -> (325.3503, -94.8501)
  line L2475 (325.3503, -94.8501) -> (325.3503, -91.8501)
  line L2476 (325.3503, -91.8501) -> (322.3503, -91.8501)
  line L2477 (322.3503, -91.8501) -> (322.3503, -88.8501)
  line L2478 (322.3503, -88.8501) -> (325.3503, -88.8501)
  line L2479 (325.3503, -88.8501) -> (325.3503, -85.8501)
  line L2480 (325.3503, -85.8501) -> (322.3503, -85.8501)
  line L2481 (322.3503, -85.8501) -> (322.3503, -82.8501)
  line L2482 (322.3503, -82.8501) -> (325.3503, -82.8501)
  line L2483 (325.3503, -82.8501) -> (325.3503, -79.8501)
  line L2484 (325.3503, -79.8501) -> (322.3503, -79.8501)
  line L2485 (322.3503, -79.8501) -> (322.3503, -76.8501)
  line L2486 (322.3503, -76.8501) -> (325.3503, -76.8501)
  line L2487 (325.3503, -76.8501) -> (325.3503, -73.8501)
  line L2488 (325.3503, -73.8501) -> (322.3503, -73.8501)
  line L2489 (322.3503, -73.8501) -> (322.3503, -70.8501)
  line L2490 (322.3503, -70.8501) -> (325.3503, -70.8501)
  line L2491 (325.3503, -70.8501) -> (325.3503, -67.8501)
  line L2492 (325.3503, -67.8501) -> (322.3503, -67.8501)
  line L2493 (322.3503, -67.8501) -> (322.3503, -64.8501)
  line L2494 (322.3503, -64.8501) -> (325.3503, -64.8501)
  line L2495 (325.3503, -64.8501) -> (325.3503, -61.8501)
  line L2496 (325.3503, -61.8501) -> (322.3503, -61.8501)
  line L2497 (322.3503, -61.8501) -> (322.3503, -58.85)
  line L2498 (322.3503, -58.85) -> (325.3503, -58.85)
  line L2499 (325.3503, -58.85) -> (325.3503, -55.85)
  line L2500 (325.3503, -55.85) -> (322.3503, -55.85)
  line L2501 (322.3503, -55.85) -> (322.3503, -52.85)
  line L2502 (322.3503, -52.85) -> (325.3503, -52.85)
  line L2503 (325.3503, -52.85) -> (325.3503, -49.85)
  line L2504 (325.3503, -49.85) -> (322.3503, -49.85)
  line L2505 (322.3503, -49.85) -> (322.3503, -46.85)
  line L2506 (322.3503, -46.85) -> (325.3503, -46.85)
  line L2507 (325.3503, -46.85) -> (325.3503, -43.85)
  line L2508 (325.3503, -43.85) -> (322.3503, -43.85)
  line L2509 (322.3503, -43.85) -> (322.3503, -40.85)
  line L2510 (322.3503, -40.85) -> (325.3503, -40.85)
  line L2511 (325.3503, -40.85) -> (325.3503, -37.85)
  line L2512 (325.3503, -37.85) -> (322.3503, -37.85)
  line L2513 (322.3503, -37.85) -> (322.3503, -34.85)
  line L2514 (322.3503, -34.85) -> (325.3503, -34.85)
  line L2515 (325.3503, -34.85) -> (325.3503, -31.85)
  line L2516 (325.3503, -31.85) -> (322.3503, -31.85)
  line L2517 (322.3503, -31.85) -> (322.3503, -28.1)
  line L2518 (322.3503, -28.1) -> (325.3503, -28.1)
  line L2519 (325.3503, -28.1) -> (325.3503, -27.35)
scale "Scale1" [no effect]
sketch "Sketch5" plane through (0, 0, 0) normal (0, 1, 0) x (1, 0, 0)
  line L0 (620.3505, -167.3501) -> (390.3505, -167.3501)
  line L1 (390.3505, -167.3501) -> (390.3505, -37.3501)
  line L2 (390.3505, -37.3501) -> (620.3505, -37.3501)
  line L3 (620.3505, -37.3501) -> (620.3505, -167.3501)
  circle A0 centre (110.4882, -152.6046) radius 2.5
  circle A1 centre (210.4882, -152.6046) radius 2.5
  circle A2 centre (110.4882, -52.6046) radius 2.5
  circle A3 centre (210.4882, -52.6046) radius 2.5
  circle A4 centre (122.9882, -140.1046) radius 2.5
  circle A5 centre (197.9882, -140.1046) radius 2.5
  circle A6 centre (122.9882, -65.1046) radius 2.5
  circle A7 centre (197.9882, -65.1046) radius 2.5
  point P0 (635.3505, -177.3501)
  dimension "d12" = 230
  dimension "d13" = 130
  dimension "d14" = 10
  dimension "d15" = 15
  dimension "d37" = 5
  dimension "d40" = 100
  dimension "d41" = 100
  dimension "d42" = 5
  dimension "d45" = 75
  dimension "d46" = 75
  dimension "d47" = 12.5
  dimension "d48" = 12.5
  measures "d12" distance of L0.start L0.end
  measures "d13" distance of L0.start L2.end
  measures "d14" distance of L0.start P0
  measures "d15" distance of L0.start P0
  measures "d37" diameter of A0
  measures "d42" diameter of A4
  measures "d47" distance of A0.centre A4.centre
  measures "d48" distance of A0.centre A4.centre
extrude "Extrude1" add sketch "Sketch4" along normal blind 3 contours L1296 L1297 L1298 L1299 L1300 L1301 L1302 L1303 L1304 L1305 L1306 L1307 L1308 L1309 L1310 L1311 L1312 L1313 L1314 L1315 L1316 L1317 L1318 L1319 L1320 L1321 L1322 L1323 L1324 L1325 L1326 L1327 L1328 L1329 L1330 L1331 L1332 L1333 L1334 L1335 L1336 L1337 L1338 L1339 L1340 L1341 L1342 L1343 L1344 L1345 L1346 L1347 L1348 L1349 L1350 L1351 L1352 L1353 L1354 L1355 L1356 L1357 L1358 L1359 L1360 L1361 L1362 L1363 L1364 L1365 L1366 L1367 L1368 L1369 L1370 L1371 L1372 L1373 L1374 L1375 L1376 L1377 L1378 L1379 L1380 L1381 L1382 L1383 L1384 L1385 L1386 L1387 L1388 L1389 L1390 L1391 L1392 L1393 L1394 L1395 L1396 L1397 L1398 L1399 L1400 L1401 L1402 L1403 L1404 L1405 L1406 L1407 L1408 L1409 L1410 L1411 L1412 L1413 L1414 L1415 L1416 L1417 L1418 L1419 L1420 L1421 L1422 L1423 L1424 L1425 L1426 L1427 L1428 L1429 L1430 L1431 L1432 L1433 L1434 L1435 L1436 L1437 L1438 L1439 L1440 L1441 L1442 L1443 L1444 L1445 L1446 L1447 L1448 L1449 L1450 L1451 L1452 L1453 L1454 L1455 L1456 L1457 L1458 L1459 L1460 L1461 L1462 L1463 L1464 L1465 L1466 L1467 L1468 L1469 L1470 L1471 L1472 L1473 L1474 L1475 L1476 L1477 L1478 L1479 L1480 L1481 L1482 L1483 L1484 L1485 L1486 L1487 L1488 L1489 L1490 L1491 L1492 L1493 L1494 L1495 L1496 L1497 L1498 L1499 L1500 L1501 L1502 L1503 L1504 L1505 L1506 L1507 L1508 L1509 L1510 L1511 L1512 L1513 L1514 L1515 L1516 L1517 L1518 L1519 L1520 L1521 L1522 L1523 L1524 L1525 L1526 L1527 L1528 L1529 L1530 L1531 L1532 L1533 L1534 L1535 L1536 L1537 L1538 L1539 L1540 L1541 L1542 L1543 L1544 L1545 L1546 L1547 L1548 L1549 L1550 L1551 L1552 L1553 L1554 L1555 L1556 L1557 L1558 L1559 L1560 L1561 L1562 L1563 L1564 L1565 L1566 L1567 L1568 L1569 L1570 L1571 L1572 L1573 L1574 L1575 L1576 L1577 L1578 L1579 L1580 L1581 L1582 L1583 L1584 L1585 L1586 L1587 L1588 L1589 L1590 L1591 L1592 L1593 L1594 L1595 L1596 L1597 L1598 L1599 L1600 L1601 L1602 L1603 L1604 L1605 L1606 L1607 L1608 L1609 L1610 L1611 L1612 L1613 L1614 L1615 L1616 L1617 L1618 L1619 L1620 L1621 L1622 L1623 L1624 L1625 L1626 L1627 L1628 L1629 L1630 L1631 L1632 L1633 L1634 L1635 L1636 L1637 L1638 L1639 L1640 L1641 L1642 L1643 L1644 L1645 L1646 L1647 L1648 L1649 L1650 L1651 L1652 L1653 L1654 L1655 L1656 L1657 L1658 L1659 L1660 L1661 L1662 L1663 L1664 L1665 L1666 L1667 L1668 L1669 L1670 L1671 L1672 L1673 L1674 L1675 L1676 L1677 L1678 L1679 L1680 L1681 L1682 L1683 L1684 L1685 L1686 L1687 L1688 L1689 L1690 L1691 L1692 L1693 L1694 L1695 L1696 L1697 L1698 L1699 L1700 L1701 L1702 L1703 L1704 L1705 L1706 L1707 L1708 L1709 L1710 L1711 L1712 L1713 L1714 L1715 L1716 L1717 L1718 L1719 L1720 L1721 L1722 L1723 L1724 L1725 L1726 L1727 L1728 L1729 L1730 L1731 L1732 L1733 L1734 L1735 L1736 L1737 L1738 L1739 L1740 L1741 L1742 L1743 L1744 L1745 L1746 L1747 L1748 L1749 L1750 L1751 L1752 L1753 L1754 L1755 L1756 L1757 L1758 L1759 L1760 L1761 L1762 L1763 L1764 L1765 L1766 L1767 L1768 L1769 L1770 L1771 L1772 L1773 L1774 L1775 L1776 L1777 L1778 L1779 L1780 L1781 L1782 L1783 L1784 L1785 L1786 L1787 L1788 L1789 L1790 L1791 L1792 L1793 L1794 L1795 L1796 L1797 L1798 L1799 L1800 L1801 L1802 L1803 L1804 L1805 L1806 L1807 L1808 L1809 L1810 L1811 L1812 L1813 L1814 L1815 L1816 L1817 L1818 L1819 L1820 L1821 L1822 L1823 L1824 L1825 L1826 L1827 L1828 L1829 L1830 L1831 L1832 L1833 L1834 L1835 L1836 L1837 L1838 L1839 L1840 L1841 L1842 L1843 L1844 L1845 L1846 L1847 L1848 L1849 L1850 L1851 L1852 L1853 L1854 L1855 L1856 L1857 L1858 L1859 L1860 L1861 L1862 L1863 L1864 L1865 L1866 L1867 L1868 L1869 L1870 L1871 L1872 L1873 L1874 L1875 L1876 L1877 L1878 L1879 L1880 L1881 L1882 L1883 L1884 L1885 L1886 L1887 L1888 L1889 L1890 L1891 L1892 L1893 L1894 L1895 L1896 L1897 L1898 L1899 L1900 L1901 L1902 L1903 L1904 L1905 L1906 L1907 L2421 L2425 L2429 L2433 L2437 L2441 L2445 L2449 L2453 L2457 L2461 L2465 L2469 L2473 L2477 L2481 L2485 L2489 L2493 L2497 L2501 L2505 L2509 L2513 L2517 makes body 1
extrude "Extrude2" add sketch "Sketch4" along normal blind 3 separate body contours L0 L1 L2 L3 L4 L5 L6 L7 L8 L9 L10 L11 L12 L13 L14 L15 L16 L17 L18 L19 L20 L21 L22 L23 L24 L25 L26 L27 L28 L29 L30 L31 L32 L33 L34 L35 L36 L37 L38 L39 L40 L41 L42 L43 L44 L45 L46 L47 L48 L49 L50 L51 L52 L53 L54 L55 L56 L57 L58 L59 L60 L61 L62 L63 L64 L65 L66 L67 L68 L69 L70 L71 L72 L73 L74 L75 L76 L77 L78 L79 L80 L81 L82 L83 L84 L85 L86 L87 L88 L89 L90 L91 L92 L93 L94 L95 L96 L97 L98 L99 L100 L101 L102 L103 L104 L105 L106 L107 L108 L109 L110 L111 L112 L113 L114 L115 L116 L117 L118 L119 L120 L121 L122 L123 L124 L125 L126 L127 L128 L129 L130 L131 L132 L133 L134 L135 L136 L137 L138 L139 L140 L141 L142 L143 L144 L145 L146 L147 L148 L149 L150 L151 L152 L153 L154 L155 L156 L157 L158 L159 L160 L161 L162 L163 L164 L165 L166 L167 L168 L169 L170 L171 L172 L173 L174 L175 L176 L177 L178 L179 L180 L181 L182 L183 L184 L185 L186 L187 L188 L189 L190 L191 L192 L193 L194 L195 L196 L197 L198 L199 L200 L201 L202 L203 L204 L205 L206 L207 L208 L209 L210 L211 L212 L213 L214 L215 L216 L217 L218 L219 L220 L221 L222 L223 L224 L225 L226 L227 L228 L229 L230 L231 L232 L233 L234 L235 L236 L237 L238 L239 L240 L241 L242 L243 L244 L245 L246 L247 L248 L249 L250 L251 L252 L253 L254 L255 L256 L257 L258 L259 L260 L261 L262 L263 L264 L265 L266 L267 L268 L269 L270 L271 L272 L273 L274 L275 L276 L277 L278 L279 L280 L281 L282 L283 L284 L285 L286 L287 L288 L289 L290 L291 L292 L293 L294 L295 L296 L297 L298 L299 L300 L301 L302 L303 L304 L305 L306 L307 L308 L309 L310 L311 L312 L313 L314 L315 L316 L317 L318 L319 L320 L321 L322 L323 L324 L325 L326 L327 L328 L329 L330 L331 L332 L333 L334 L335 L336 L337 L338 L339 L340 L341 L342 L343 L344 L345 L346 L347 L348 L349 L350 L351 L352 L353 L354 L355 L356 L357 L358 L359 L360 L361 L362 L363 L364 L365 L366 L367 L368 L369 L370 L371 L372 L373 L374 L375 L376 L377 L378 L379 L380 L381 L382 L383 L384 L385 L386 L387 L388 L389 L390 L391 L392 L393 L394 L395 L396 L397 L398 L399 L400 L401 L402 L403 L404 L405 L406 L407 L408 L409 L410 L411 L412 L413 L414 L415 L416 L417 L418 L419 L420 L421 L422 L423 L424 L425 L426 L427 L847 L851 L855 makes body 2
extrude "Extrude3" add sketch "Sketch4" along normal blind 3 separate body contours L205 L209 L213 L428 L429 L430 L431 L432 L433 L434 L435 L436 L437 L438 L439 L440 L441 L442 L443 L444 L445 L446 L447 L448 L449 L450 L451 L452 L453 L454 L455 L456 L457 L458 L459 L460 L461 L462 L463 L464 L465 L466 L467 L468 L469 L470 L471 L472 L473 L474 L475 L476 L477 L478 L479 L480 L481 L482 L483 L484 L485 L486 L487 L488 L489 L490 L491 L492 L493 L494 L495 L496 L497 L498 L499 L500 L501 L502 L503 L504 L505 L506 L507 L508 L509 L510 L511 L512 L513 L514 L515 L516 L517 L518 L519 L520 L521 L522 L523 L524 L525 L526 L527 L528 L529 L530 L531 L532 L533 L534 L535 L536 L537 L538 L539 L540 L541 L542 L543 L544 L545 L546 L547 L548 L549 L550 L551 L552 L553 L554 L555 L556 L557 L558 L559 L560 L561 L562 L563 L564 L565 L566 L567 L568 L569 L570 L571 L572 L573 L574 L575 L576 L577 L578 L579 L580 L581 L582 L583 L584 L585 L586 L587 L588 L589 L590 L591 L592 L593 L594 L595 L596 L597 L598 L599 L600 L601 L602 L603 L604 L605 L606 L607 L608 L609 L610 L611 L612 L613 L614 L615 L616 L617 L618 L619 L620 L621 L622 L623 L624 L625 L626 L627 L628 L629 L630 L631 L632 L633 L634 L635 L636 L637 L638 L639 L640 L641 L642 L643 L644 L645 L646 L647 L648 L649 L650 L651 L652 L653 L654 L655 L656 L657 L658 L659 L660 L661 L662 L663 L664 L665 L666 L667 L668 L669 L670 L671 L672 L673 L674 L675 L676 L677 L678 L679 L680 L681 L682 L683 L684 L685 L686 L687 L688 L689 L690 L691 L692 L693 L694 L695 L696 L697 L698 L699 L700 L701 L702 L703 L704 L705 L706 L707 L708 L709 L710 L711 L712 L713 L714 L715 L716 L717 L718 L719 L720 L721 L722 L723 L724 L725 L726 L727 L728 L729 L730 L731 L732 L733 L734 L735 L736 L737 L738 L739 L740 L741 L742 L743 L744 L745 L746 L747 L748 L749 L750 L751 L752 L753 L754 L755 L756 L757 L758 L759 L760 L761 L762 L763 L764 L765 L766 L767 L768 L769 L770 L771 L772 L773 L774 L775 L776 L777 L778 L779 L780 L781 L782 L783 L784 L785 L786 L787 L788 L789 L790 L791 L792 L793 L794 L795 L796 L797 L798 L799 L800 L801 L802 L803 L804 L805 L806 L807 L808 L809 L810 L811 L812 L813 L814 L815 L816 L817 L818 L819 L820 L821 L822 L823 L824 L825 L826 L827 L828 L829 L830 L831 L832 L833 L834 L835 L836 L837 L838 L839 L840 L841 L842 L843 L844 L845 L846 L847 L848 L849 L850 L851 L852 L853 L854 L855 makes body 3
extrude "Extrude4" add sketch "Sketch4" along normal blind 3 separate body contours L856 L857 L858 L859 L860 L861 L862 L863 L864 L865 L866 L867 L868 L869 L870 L871 L872 L873 L874 L875 L876 L877 L878 L879 L880 L881 L882 L883 L884 L885 L886 L887 L888 L889 L890 L891 L892 L893 L894 L895 L896 L897 L898 L899 L900 L901 L902 L903 L904 L905 L906 L907 L908 L909 L910 L911 L912 L913 L914 L915 L916 L917 L918 L919 L920 L921 L922 L923 L924 L925 L926 L927 L928 L929 L930 L931 L932 L933 L934 L935 L936 L937 L938 L939 L940 L941 L942 L943 L944 L945 L946 L947 L948 L949 L950 L951 L952 L953 L954 L955 L956 L957 L958 L959 L960 L961 L962 L963 L964 L965 L966 L967 L968 L969 L970 L971 L972 L973 L974 L975 L976 L977 L978 L979 L980 L981 L982 L983 L984 L985 L986 L987 L988 L989 L990 L991 L992 L993 L994 L995 L996 L997 L998 L999 L1000 L1001 L1002 L1003 L1004 L1005 L1006 L1007 L1008 L1009 L1010 L1011 L1012 L1013 L1014 L1015 L1016 L1017 L1018 L1019 L1020 L1021 L1022 L1023 L1024 L1025 L1026 L1027 L1028 L1029 L1030 L1031 L1032 L1033 L1034 L1035 L1036 L1037 L1038 L1039 L1040 L1041 L1042 L1043 L1044 L1045 L1046 L1047 L1048 L1049 L1050 L1051 L1052 L1053 L1054 L1055 L1056 L1057 L1058 L1059 L1060 L1061 L1062 L1063 L1064 L1065 L1066 L1067 L1068 L1069 L1070 L1071 L1072 L1073 L1074 L1075 L1076 L1080 L1084 L1088 L1092 L1096 L1100 L1104 L1108 L1112 L1116 L1120 L1124 L1128 L1132 L1136 L1140 L1144 L1148 L1152 L1156 L1160 L1164 L1168 L1172 L1176 makes body 4